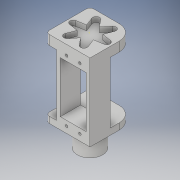
# Autodesk Inventor part: Pata - Hombro
Saved by Autodesk Inventor 2019 (Build 230136000, 136)
## iProperties
Created: 2020-03-08
Part Number: Pata - Hombro
Material: Genérico
Document SubType Name: Modeling
Designer: eddysanoli
Density: 1 g/cm^3
Appearance: Valor por defecto
ancho_servo: 20.500 mm
largo_servo: 40.500 mm
diametro_eje_hombro: 20.000 mm
profundidad_hombro: 35.094 mm
Author: eddysanoli
Autodesk Inventor part; units mm, degrees
ref_plane "YZ Plane" through (0, 0, 0) normal (1, 0, 0) x (0, 1, 0)
ref_plane "XZ Plane" through (0, 0, 0) normal (0, 1, 0) x (-1, 0, 0)
ref_plane "XY Plane" through (0, 0, 0) normal (0, 0, 1) x (1, 0, 0)
sketch "Boceto1" plane through (0, 0, 0) normal (0, 1, 0) x (-1, 0, 0)
  circle A0 centre (0, 0) radius 7.45 construction
  line L0 (0, 7.45) -> (4.6066, 13.113)
  arc A1 (9.0529, 10.5459) -> (4.6066, 13.113) centre (6.6235, 11.4723) ccw
  line L1 (9.0529, 10.5459) -> (6.4519, 3.725)
  line L2 (6.4519, 3.725) -> (13.6595, 2.5671)
  arc A2 (13.6595, -2.5671) -> (13.6595, 2.5671) centre (13.2471, 0) ccw
  line L3 (13.6595, -2.5671) -> (6.4519, -3.725)
  line L4 (6.4519, -3.725) -> (9.0529, -10.5459)
  arc A3 (4.6066, -13.113) -> (9.0529, -10.5459) centre (6.6235, -11.4723) ccw
  line L5 (4.6066, -13.113) -> (0, -7.45)
  line L6 (0, -7.45) -> (-4.6066, -13.113)
  arc A4 (-9.0529, -10.5459) -> (-4.6066, -13.113) centre (-6.6235, -11.4723) ccw
  line L7 (-9.0529, -10.5459) -> (-6.4519, -3.725)
  line L8 (-6.4519, -3.725) -> (-13.6595, -2.5671)
  arc A5 (-13.6595, 2.5671) -> (-13.6595, -2.5671) centre (-13.2471, 0) ccw
  line L9 (-13.6595, 2.5671) -> (-6.4519, 3.725)
  line L10 (-6.4519, 3.725) -> (-9.0529, 10.5459)
  line L11 (0, 7.45) -> (-4.6066, 13.113)
  arc A6 (-4.6066, 13.113) -> (-9.0529, 10.5459) centre (-6.6235, 11.4723) ccw
  dimension "d6" = 14.9
  dimension "d11" = 2.6
  dimension "d12" = 7.3
  dimension "d13" = 60
  constraints: 24 end point, 18 point on circle, 12 tangent, 11 equal length, 7 centre point, 5 equal radius, 4 vertical alignment, 2 coincident, 2 horizontal alignment
  measures "d6" diameter of A0
  measures "d11" radius of A6
  measures "d12" distance of L9.end L10.end
sketch "Boceto2" plane through (0, 0, 0) normal (0, 1, 0) x (-1, 0, 0)
  line L0 (17.5471, 17.5471) -> (-17.5471, 17.5471)
  line L1 (-17.5471, 17.5471) -> (-17.5471, -17.5471)
  line L2 (-17.5471, -17.5471) -> (17.5471, -17.5471)
  line L3 (17.5471, -17.5471) -> (17.5471, 17.5471)
  arc A0 (-13.6595, 2.5671) -> (-13.6595, -2.5671) centre (-13.2471, 0) ccw projected
  point P0 (0, 0)
  point P1 (0, -17.5471)
  point P2 (17.5471, 0)
  dimension "d14" = 4.3
  dimension "profundidad_hombro" = 35.0941
  constraints: 8 end point, 2 midpoint, 2 parallel, 2 perpendicular, 1 horizontal, 1 horizontal alignment, 1 vertical alignment
  measures "d14" distance from line of L1 A0.centre
  measures "profundidad_hombro" distance of L0.end L1.end
extrude "Extrusión1" add sketch "Boceto2" against normal blind 7.55
extrude "Extrusión2" cut sketch "Boceto1" against normal blind 4
sketch "Boceto3" plane through (0, -7.55, 0) normal (0, -1, 0) x (1, 0, 0)
  line L0 (17.5471, -17.5471) -> (-17.5471, -17.5471) construction
  line L1 (-8.9529, 17.5471) -> (17.5471, 17.5471)
  line L2 (17.5471, 17.5471) -> (17.5471, 1.5471)
  line L3 (17.5471, 1.5471) -> (-8.9529, 1.5471)
  line L4 (-8.9529, 1.5471) -> (-8.9529, 17.5471)
  line L5 (17.5471, 17.5471) -> (-17.5471, 17.5471) projected
  line L6 (17.5471, 17.5471) -> (-17.5471, 17.5471) projected
  line L7 (-17.5471, 17.5471) -> (-17.5471, -17.5471) projected
  line L8 (-17.5471, -17.5471) -> (17.5471, -17.5471) projected
  line L9 (17.5471, -17.5471) -> (17.5471, 17.5471) projected
  point P0 (0, 0)
  point P1 (-2.8923, 1.5471)
  dimension "d20" = 16
  dimension "d59" = 26.5
  constraints: 8 end point, 3 perpendicular, 2 point on line
  measures "d20" distance of L1.end L2.end
  measures "d59" distance of L2.end L3.end
extrude "Extrusión3" add sketch "Boceto3" along normal blind 48.5 contours L1 L2 L3 L4
sketch "Boceto4" plane through (0, -56.05, 0) normal (0, -1, 0) x (1, 0, 0)
  line L0 (17.5471, 17.5471) -> (17.5471, -17.5471) projected
  line L1 (-17.5471, -17.5471) -> (17.5471, -17.5471)
  line L2 (17.5471, -17.5471) -> (17.5471, 17.5471)
  line L3 (17.5471, 17.5471) -> (-17.5471, 17.5471)
  line L4 (-17.5471, 17.5471) -> (-17.5471, -17.5471)
  point P0 (0, 0)
  constraints: 8 end point, 2 parallel, 1 horizontal, 1 perpendicular
extrude "Extrusión4" add sketch "Boceto4" along normal blind 5
sketch "Boceto5" plane through (0, -61.05, 0) normal (0, -1, 0) x (1, 0, 0)
  circle A0 centre (0, 0) radius 10
  dimension "diametro_eje_hombro" = 20
  constraints: 1 centre point, 1 coincident
  measures "diametro_eje_hombro" diameter of A0
extrude "Extrusión5" add sketch "Boceto5" along normal blind 18
sketch "Sketch11" plane through (-17.5471, 0, 17.5471) normal (0, 0, 1) x (1, 0, 0)
  line L0 (11.5941, -52.05) -> (32.0941, -52.05)
  line L1 (32.0941, -52.05) -> (32.0941, -11.55)
  line L2 (32.0941, -11.55) -> (11.5941, -11.55)
  line L3 (11.5941, -11.55) -> (11.5941, -52.05)
  line L4 (8.5941, -7.55) -> (8.5941, -56.05) projected
  line L5 (35.0941, 0) -> (35.0941, -61.05) projected
  point P0 (17.5471, 0)
  point P1 (11.5941, -31.8)
  point P2 (8.5941, -31.8)
  dimension "d60" = 40.5
  dimension "d61" = 3
  dimension "d62" = 3
  constraints: 8 end point, 2 midpoint, 2 parallel, 1 horizontal, 1 horizontal alignment, 1 perpendicular
  measures "d60" distance of L2.end L0.start
  measures "d61" distance between parallel lines of L4 L3
  measures "d62" distance between parallel lines of L5 L1
extrude "Extrusion12" cut sketch "Sketch11" against normal up to surface (16 mm away)
sketch "Sketch12" plane through (-17.5471, 0, 17.5471) normal (0, 0, 1) x (1, 0, 0)
  circle A0 centre (16.5941, -56) radius 1
  circle A1 centre (27.0941, -56) radius 1
  circle A2 centre (27.0941, -7.6) radius 1
  circle A3 centre (16.5941, -7.6) radius 1
  line L0 (32.0941, -52.05) -> (11.5941, -52.05) projected
  line L1 (11.5941, -11.55) -> (32.0941, -11.55) projected
  line L2 (32.0941, -11.55) -> (32.0941, -52.05) projected
  line L3 (11.5941, -52.05) -> (11.5941, -11.55) projected
  point P0 (17.5471, 0)
  dimension "d65" = 2
  dimension "d66" = 3.95
  dimension "d67" = 3.95
  dimension "d68" = 5
  dimension "d69" = 5
  constraints: 4 centre point, 3 equal radius, 2 horizontal alignment, 2 vertical alignment
  measures "d65" diameter of A0
  measures "d66" distance from line of L0 A0.centre
  measures "d67" distance from line of L1 A3.centre
  measures "d68" distance from line of L2 A2.centre
  measures "d69" distance from line of L3 A0.centre
extrude "Extrusion13" cut sketch "Sketch12" against normal blind 14 contours A0 | A1 | A2 | A3
fillet "Fillet2" radius 12 2 edges at (17.5471, -3.775, -17.5471) (17.5471, -58.55, -17.5471)
fillet "Fillet3" radius 3 5 edges at (-10, -61.05, 0) (-17.5471, -58.55, 17.5471) (-17.5471, -3.775, 17.5471) (-17.5471, -3.775, -17.5471) (-17.5471, -58.55, -17.5471)
equation "\"d6\" = diametro_aspa"
equation "\"d11\" = diametro_petalo"
equation "\"d12\" = largo_petalo"
equation "\"d62\" = d61"
equation "\"d67\" = d66"
equation "\"diametro_aspa\" = 14.9"
equation "\"diametro_petalo\" = 2.6"
equation "\"largo_petalo\" = 7.3"
